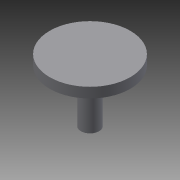
# Autodesk Inventor part: Fixture_Knob_2
Saved by Autodesk Inventor 2015 (Build 190159000, 159)
## iProperties
Created: 2014-12-16
Part Number: Fixture_Knob_2
Material: Generic
Document SubType Name: Modeling
Designer: amarschn
Density: 1 g/cm^3
Appearance: Default
Author: amarschn
Autodesk Inventor part; units mm, degrees
ref_plane "YZ Plane" through (0, 0, 0) normal (1, 0, 0) x (0, 1, 0)
ref_plane "XZ Plane" through (0, 0, 0) normal (0, 1, 0) x (-1, 0, 0)
ref_plane "XY Plane" through (0, 0, 0) normal (0, 0, 1) x (1, 0, 0)
sketch "Sketch1" plane through (0, 0, 0) normal (1, 0, 0) x (0, 1, 0)
  line L0 (0, 0) -> (0, -25.4)
  line L1 (0, -25.4) -> (-6.35, -25.4)
  line L2 (-6.35, -25.4) -> (-6.35, -8.89)
  line L3 (-13.97, -5.715) -> (-39.37, -5.715)
  line L4 (-39.37, -5.715) -> (-39.37, 0)
  line L5 (-39.37, 0) -> (0, 0)
  line L6 (-6.35, -8.89) -> (-13.97, -8.89)
  line L7 (-13.97, -8.89) -> (-13.97, -5.715)
  dimension "d0" = 6.35
  dimension "d2" = 7.62
  dimension "d3" = 25.4
  dimension "d4" = 25.4
  dimension "d5" = 5.715
  dimension "d6" = 8.89
  constraints: 16 end point, 6 perpendicular, 1 horizontal, 1 vertical
  measures "d0" distance of L0.end L1.end
  measures "d2" distance between parallel lines of L7 L2
  measures "d3" distance of L3.start L3.end
  measures "d4" distance of L0.start L0.end
  measures "d5" distance of L3.end L4.end
  measures "d6" distance between parallel lines of L5 L6
revolve "Revolution1" add sketch "Sketch1" angle 360 about axis through (0, -39.37, 0) along (0, 1, 0)
body "Solid1"
